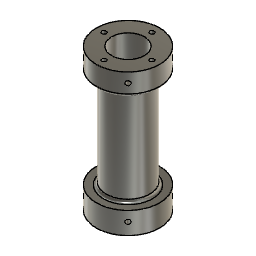
Engine Block Pioneer v4 (Autodesk Fusion 360 design; units mm, degrees)
Autodesk Fusion 360 part; units mm, degrees
sketch "Schizzo1" plane through (0, 0, 0) normal (0, 0, 1) x (1, 0, 0)
  circle A0 centre (0, 0) radius 29
  circle A1 centre (0, 0) radius 15
  circle A2 centre (0, 0) radius 20
  dimension "d1" = 58
  constraint coincident A0.centre A1.centre
  constraint concentric A0 A1
  constraint concentric A1 A2
  measures "d1" diameter of A0
extrude "Estrusione1" add sketch "Schizzo1" along normal blind 20 contours A0 | A2
ref_plane "Piano di lavoro1" through (0, 0, 20) normal (0, 0, 1) x (1, 0, 0)
sketch "Schizzo2" plane through (0, 0, 20) normal (0, 0, 1) x (1, 0, 0)
  circle A0 centre (0, 0) radius 20
  dimension "d5" = 40
  constraint coincident A0.centre origin
  measures "d5" diameter of A0
sketch "Schizzo3" plane through (0, 0, 20) normal (0, 0, 1) x (1, 0, 0)
  circle A0 centre (0, 0) radius 15
  constraint coincident A0.centre origin
ref_plane "Piano di lavoro2" through (0, 0, 20) normal (0, 0, 1) x (1, 0, 0)
sketch "Schizzo4" plane through (0, 0, 20) normal (0, 0, 1) x (1, 0, 0)
  circle A0 centre (0, 0) radius 15
  circle A1 centre (0, 0) radius 20
  constraint coincident A0.centre A1.centre
extrude "Estrusione2" add sketch "Schizzo4" along normal blind 90
ref_plane "Piano di lavoro3" through (0, 0, 110) normal (0, 0, 1) x (1, 0, 0)
sketch "Schizzo5" plane through (0, 0, 110) normal (0, 0, 1) x (1, 0, 0)
  circle A0 centre (0, 0) radius 29
  dimension "d10" = 58
  constraint coincident A0.centre origin
  measures "d10" diameter of A0
sketch "Schizzo6" plane through (0, 0, 110) normal (0, 0, 1) x (1, 0, 0)
  circle A0 centre (0, 0) radius 15
  constraint coincident A0.centre origin
ref_plane "Piano di lavoro4" through (0, 0, 110) normal (0, 0, 1) x (1, 0, 0)
sketch "Schizzo7" plane through (0, 0, 110) normal (0, 0, 1) x (1, 0, 0)
  circle A0 centre (0, 0) radius 15
  circle A1 centre (0, 0) radius 29
  dimension "d12" = 58
  constraint coincident A0.centre A1.centre
  measures "d12" diameter of A1
extrude "Estrusione3" add sketch "Schizzo7" along normal blind 20
fillet "Raccordo1" radius 2.5 1 edges at (-27.0375, -10.4868, 110) 1 faces at (-19.9006, 1.9914, 80)
sketch "Schizzo8" plane through (0, 0, 0) normal (1, 0, 0) x (0, 1, 0)
ref_plane "Piano di lavoro5" through (0, 0, 130) normal (0, 0, 1) x (1, 0, 0)
sketch "Schizzo9" plane through (0, 0, 130) normal (0, 0, 1) x (1, 0, 0)
  point P0 (0, 22)
  point P1 (22, 0)
  point P2 (-22, 0)
  point P3 (0, -22)
ref_plane "Piano di lavoro6" through (0, 0, 0) normal (0, 0, -1) x (-1, 0, 0)
sketch "Schizzo10" plane through (0, 0, 0) normal (0, 0, -1) x (-1, 0, 0)
  point P0 (0, -22)
  point P1 (-22, 0)
  point P2 (22, 0)
  point P3 (0, 22)
hole "Foratura1" at (-22, 0, 0) direction (0, 0, 1) diameter 4 depth 15 tip angle 118
hole "Foratura2" at (0.0055, 22.0041, 0) direction (0, 0, 1) diameter 4 depth 15 tip angle 118
hole "Foratura3" at (22.0297, 0.0064, 0) direction (0, 0, 1) diameter 4 depth 15 tip angle 118
hole "Foratura4" at (0.0297, -21.9985, 0) direction (0, 0, 1) diameter 4 depth 15 tip angle 118
hole "Foratura5" at (0, -22, 130) direction (0, 0, -1) diameter 4 depth 15 tip angle 118
ref_plane "Piano di lavoro7" through (0, 0, 130) normal (0, 0, 1) x (1, 0, 0)
sketch "Schizzo11" plane through (0, 0, 130) normal (0, 0, 1) x (1, 0, 0)
  point P0 (0, 22)
  point P1 (22, 0)
  point P2 (-22, 0)
hole "Foratura6" at (0, 22, 130) direction (0, 0, -1) diameter 4 depth 15 tip angle 118
sketch "Schizzo12" plane through (0, 0, 130) normal (0, 0, 1) x (-1, 0, 0)
  circle A0 centre (0, -22) radius 2
  circle A1 centre (0, 22) radius 2
  circle A2 centre (0, 0) radius 15
  circle A3 centre (0, 0) radius 29
  point P0 (-22, 0)
hole "Foratura7" at (22, 0, 130) direction (0, 0, -1) diameter 4 depth 15 tip angle 118
sketch "Schizzo13" plane through (0, 0, 130) normal (0, 0, 1) x (-1, 0, 0)
  circle A0 centre (-22, 0) radius 2
  circle A1 centre (0, -22) radius 2
  circle A2 centre (0, 22) radius 2
  circle A3 centre (0, 0) radius 15
  circle A4 centre (0, 0) radius 29
  point P0 (22, 0)
hole "Foratura8" at (-22, 0, 130) direction (0, 0, -1) diameter 4 depth 15 tip angle 118
hole "Foratura9" at (20.5061, -20.5061, 120) direction (-0.707107, 0.707107, 0) diameter 4 depth 15 tip angle 118
delete_face "EliminaFaccia1" 1 faces at (17.8158, -16.5712, 118.204)
hole "Foratura10" at (20.5061, -20.5061, 121) direction (-0.707107, 0.707107, 0) diameter 4 depth 12 tip angle 118
hole "Foratura11" at (20.5061, 20.5061, 121) direction (-0.707107, -0.707107, 0) diameter 4 depth 12 tip angle 118
hole "Foratura12" at (-22.2153, 18.6408, 121) direction (0.766044, -0.642788, 0) diameter 4 depth 12 tip angle 118
hole "Foratura13" at (-20.5061, -20.5061, 121) direction (0.707107, 0.707107, 0) diameter 4 depth 12 tip angle 118
form "Forma1" [no effect]
hole "Foratura14" at (20.5061, -20.5061, 11) direction (-0.707107, 0.707107, 0) diameter 4 depth 12 tip angle 118
hole "Foratura15" at (20.5061, 20.5061, 11) direction (-0.707107, -0.707107, 0) diameter 4 depth 12 tip angle 118
hole "Foratura16" at (-20.5061, 20.5061, 11) direction (0.707107, -0.707107, 0) diameter 4 depth 12 tip angle 118
hole "Foratura17" at (-20.5061, -20.5061, 11) direction (0.707107, 0.707107, 0) diameter 4 depth 12 tip angle 118
